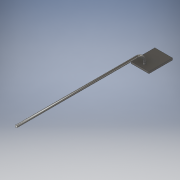
# Autodesk Inventor part: vent cover
Saved by Autodesk Inventor 2017 (Build 210142000, 142)
## iProperties
Created: 2017-06-23
Part Number: vent cover
Material: Generic
Document SubType Name: Modeling
Designer: cas7
Density: 1 g/cm^3
Appearance: Default
Author: cas7
Autodesk Inventor part; units mm, degrees
ref_plane "YZ Plane" through (0, 0, 0) normal (1, 0, 0) x (0, 1, 0)
sketch "Sketch1" plane through (0, 0, 0) normal (0, 1, 0) x (-1, 0, 0)
  line L0 (0, 0) -> (150, 0)
  line L1 (150, 0) -> (150, -200)
  line L2 (150, -200) -> (0, -200)
  line L3 (0, -200) -> (0, 0)
  dimension "d0" = 150
  dimension "d1" = 200
  constraints: 8 end point, 2 parallel, 1 horizontal, 1 perpendicular
  measures "d0" distance of L1.end L2.end
  measures "d1" distance of L0.end L1.end
extrude "Extrusion1" add sketch "Sketch1" along normal blind 15
sketch "Sketch2" plane through (0, 15, 0) normal (0, 1, 0) x (1, 0, 0)
  circle A0 centre (-75, 38.1) radius 10
  line L0 (-150, 0) -> (0, 0) projected
  line L1 (0, 0) -> (-150, 0)
  line L2 (-181.75, -31.75) -> (31.75, -31.75)
  dimension "d5" = 20
  dimension "d15" = 31.75
  constraints: 4 end point, 1 centre point, 1 collinear
  measures "d5" diameter of A0
  measures "d15" distance between parallel lines of L0 L2
ref_plane "Work Plane2" through (0, 15, 0) normal (0, 0, 1) x (1, 0, 0)
ref_plane "Work Plane3" through (-150, 0, 50.8) normal (0, 0, 1) x (1, 0, 0)
ref_plane "Work Plane5" through (0, 15, 31.75) normal (0, 0, 1) x (1, 0, 0)
revolve "Revolution2" add sketch "Sketch2" angle 90 about axis through (-181.75, 15, 31.75) along (1, 0, 0)
sketch "Sketch7" plane through (-75, 84.85, 31.75) normal (0, 0, 1) x (1, 0, 0)
  circle A0 centre (0, 0) radius 10 projected
  point P0 (75, -84.85)
extrude "Extrusion3" add sketch "Sketch7" along normal blind 1016
sketch "Sketch8" plane through (0, 15, 0) normal (0, 1, 0) x (1, 0, 0)
  circle A0 centre (-75, 38.1) radius 10 projected
  line L0 (-150, 0) -> (0, 0) projected
  line L1 (0, 0) -> (0, 200) projected
  line L2 (0, 200) -> (-150, 200) projected
  line L3 (-150, 200) -> (-150, 0) projected
extrude "Extrusion4" add sketch "Sketch8" against normal blind 30.0228
sketch "Sketch9" plane through (0, 15, 0) normal (0, 1, 0) x (1, 0, 0)
  circle A0 centre (-75, 38.1) radius 10 projected
  line L0 (-150, 0) -> (0, 0) projected
  line L1 (0, 0) -> (0, 200) projected
  line L2 (0, 200) -> (-150, 200) projected
  line L3 (-150, 200) -> (-150, 0) projected
extrude "Extrusion5" cut sketch "Sketch9" against normal blind 15.0114
body "Solid1"
